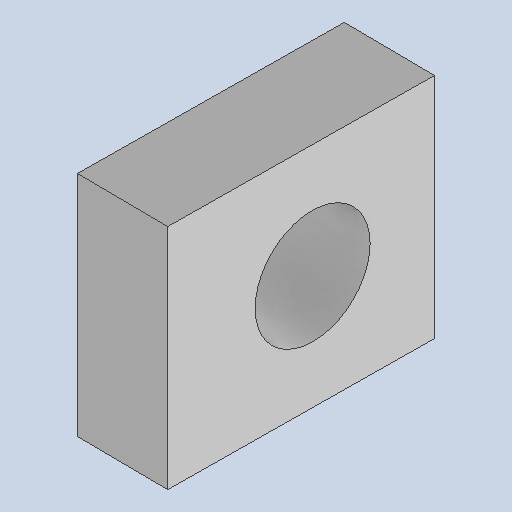
# Autodesk Inventor part: seilatrappeHalterMini
Saved by Autodesk Inventor 2025 (Build 290162010, 162A)
## iProperties
Created: 2024-11-20
Part Number: seilatrappeHalterMini
Material: OHNE_Pseudo-Teil
Document SubType Name: Modeling
Designer: Admin
Density: 1 g/cm^3
Appearance: Vorgabe(2)
Author: Admin
Autodesk Inventor part; units mm, degrees
ref_plane "YZ Plane" through (0, 0, 0) normal (1, 0, 0) x (0, 1, 0)
ref_plane "XZ Plane" through (0, 0, 0) normal (0, 1, 0) x (-1, 0, 0)
ref_plane "XY Plane" through (0, 0, 0) normal (0, 0, 1) x (1, 0, 0)
sketch "Skizze1" plane through (0, 0, 0) normal (0, 0, 1) x (1, 0, 0)
  line L0 (-1.9683, -1.568) -> (-1.9393, 1.4318) projected
  line L1 (-1.9683, -1.568) -> (2.0315, -1.6068) projected
  line L2 (2.0606, 1.3931) -> (2.0315, -1.6068) projected
  line L3 (2.0509, 0.3931) -> (-1.9489, 0.4319)
  line L4 (-2.0614, -11.1676) -> (-2.0323, -8.1677) projected
  line L5 (-2.0614, -11.1676) -> (1.9384, -11.2063) projected
  line L6 (1.9675, -8.2065) -> (1.9384, -11.2063) projected
  line L7 (1.9675, -8.2065) -> (-2.0323, -8.1677) projected
  point P0 (0, 0)
  dimension "d11" = 1
  constraints: 2 end point, 2 point on line
  measures "d11" distance from line of L2.start L3
extrude "Extrusion1" add sketch "Skizze1" along normal blind 10
sketch "Skizze2" plane through (-2.0323, -8.1677, 0) normal (0.0096951, 0.999953, 0) x (0.999953, -0.0096951, 0)
  line L0 (4, 0) -> (0, 0) projected
  line L1 (0, 0) -> (0, -10) projected
  line L2 (4, -10) -> (0, -10) projected
  line L3 (4, 0) -> (4, -10) projected
  point P0 (1.953, 0)
extrude "Extrusion2" add sketch "Skizze2" along normal through all
sketch "Skizze3" plane through (-2.0614, -11.1676, 0) normal (-0.999953, 0.0096951, 0) x (0, 0, 1)
  arc A0 (5, 8.3) -> (5, 4.3) centre (5, 6.3) ccw
  point P0 (0, 11.187)
  constraints: 2 point on circle, 1 centre point, 4 other
hole "Bohrung1" at (-2.0003, -4.8679, 5) direction (0.999953, -0.0096951, 0) diameter 5 end through all
